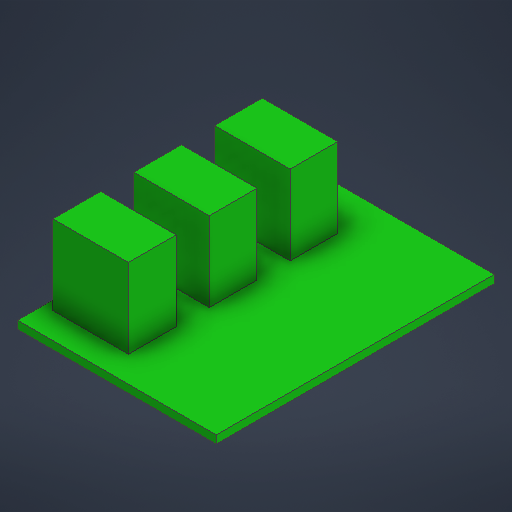
# Autodesk Inventor part: temp_pcb
Saved by Autodesk Inventor 2026.1 (Build 301233000, 233)
## iProperties
Created: 2025-09-25
Part Number: temp_pcb
Material: Generic
Document SubType Name: Modeling
Designer: emanuel
Density: 1 g/cm^3
Appearance: Default
Author: emanuel
Autodesk Inventor part; units mm, degrees
ref_plane "YZ Plane" through (0, 0, 0) normal (1, 0, 0) x (0, 1, 0)
ref_plane "XZ Plane" through (0, 0, 0) normal (0, 1, 0) x (-1, 0, 0)
ref_plane "XY Plane" through (0, 0, 0) normal (0, 0, 1) x (1, 0, 0)
sketch "Sketch1" plane through (0, 0, 0) normal (0, 1, 0) x (-1, 0, 0)
  line L0 (0, 0) -> (50, 0)
  line L1 (50, 0) -> (50, -70)
  line L2 (50, -70) -> (0, -70)
  line L3 (0, -70) -> (0, 0)
  dimension "d0" = 50
  dimension "d1" = 70
  constraints: 8 end point, 2 parallel, 1 horizontal, 1 perpendicular
  measures "d0" distance of L1.end L2.end
  measures "d1" distance of L0.end L1.end
extrude "Extrusion1" add sketch "Sketch1" along normal blind 2
sketch "Sketch2" plane through (0, 2, 0) normal (0, 1, 0) x (1, 0, 0)
  line L0 (-47.6458, 6.5409) -> (-28.6458, 6.5409)
  line L1 (-28.6458, 6.5409) -> (-28.6458, 18.5409)
  line L2 (-28.6458, 18.5409) -> (-47.6458, 18.5409)
  line L3 (-47.6458, 18.5409) -> (-47.6458, 6.5409)
  line L4 (-47.6458, 26.8862) -> (-28.6458, 26.8862)
  line L5 (-28.6458, 26.8862) -> (-28.6458, 38.8862)
  line L6 (-28.6458, 38.8862) -> (-47.6458, 38.8862)
  line L7 (-47.6458, 38.8862) -> (-47.6458, 26.8862)
  line L8 (-47.6458, 47.2315) -> (-28.6458, 47.2315)
  line L9 (-28.6458, 47.2315) -> (-28.6458, 59.2315)
  line L10 (-28.6458, 59.2315) -> (-47.6458, 59.2315)
  line L11 (-47.6458, 59.2315) -> (-47.6458, 47.2315)
  point P0 (0, 0)
  dimension "d4" = 19
  dimension "d5" = 12
  dimension "d6" = 19
  dimension "d7" = 12
  dimension "d8" = 19
  dimension "d9" = 12
  constraints: 24 end point, 6 parallel, 3 horizontal, 3 perpendicular, 2 point on line
  measures "d4" distance of L2.end L1.end
  measures "d5" distance of L1.end L0.end
  measures "d6" distance of L6.end L5.end
  measures "d7" distance of L5.end L4.end
  measures "d8" distance of L10.end L9.end
  measures "d9" distance of L9.end L8.end
extrude "Extrusion2" add sketch "Sketch2" along normal blind 20
body "Solid1"
